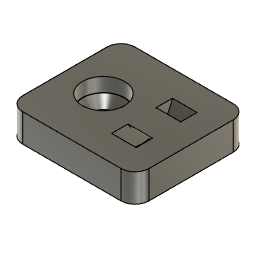
2020 Zip Tie Mount v5 (Autodesk Fusion 360 design; units mm, degrees)
Autodesk Fusion 360 part; units mm, degrees
note: some values were not read from the file. Set by a fixed rule: which sketch regions a step uses.
sketch "Sketch1" plane through (0, 0, 0) normal (0, 0, 1) x (1, 0, 0)
  line L0 (9, 8) -> (-9, 8)
  line L1 (-9, 8) -> (-9, -8)
  line L2 (-9, -8) -> (9, -8)
  line L3 (9, -8) -> (9, 8)
  circle A0 centre (-3.5, 0) radius 1.75
  circle A1 centre (-3.5, 0) radius 3
  line L4 (9, -2.8) -> (-9, -2.8)
  line L5 (-9, -2.8) -> (-9, 2.8)
  line L6 (-9, 2.8) -> (9, 2.8)
  line L7 (9, 2.8) -> (9, -2.8)
  line L8 (9, -2.8) -> (-9, 2.8) construction
  line L9 (-9, -2.8) -> (9, 2.8) construction
  dimension "d1" = 18
  dimension "d2" = 16
  dimension "d5" = 3.5
  dimension "d6" = 6
  dimension "d9" = 5.6
  dimension "d12" = 3.5
  dimension "d23" = 8
  constraint horizontal L0
  constraint perpendicular L0 L1
  constraint parallel L0 L2
  constraint parallel L1 L3
  constraint concentric A0 A1
  constraint horizontal L4
  constraint perpendicular L4 L5
  constraint parallel L4 L6
  constraint parallel L5 L7
  constraint coincident L3 L4.start
  constraint coincident L8 origin
  constraint coincident L9 origin
  constraint horizontal origin A0.centre
  constraint coincident L1 L4.end
  measures "d1" distance of L1.end L2.end
  measures "d2" distance of L0.end L1.end
  measures "d5" diameter of A0
  measures "d6" diameter of A1
  measures "d9" distance of L4 L6
  measures "d12" distance of origin A0.centre
  measures "d23" distance of L0 A0.centre
extrude "Extrude1" add sketch "Sketch1" along normal blind 2
extrude "Extrude2" add sketch "Sketch1" along normal blind 4 contours L0 L1 L3 A1 L6 | L3 A1 L4 L6 L7 | L1 A1 L4 L5 L6 | L1 L2 L3 A1 L4
extrude "Extrude3" add sketch "Sketch1" against normal blind 1 contours L3 A1 L4 L6 L7 | L1 A1 L4 L5 L6 | A1 L4 L6
sketch "Sketch2" plane through (9, 0, 0) normal (1, 0, 0) x (0, 1, 0)
  line L0 (-8, 0) -> (-2.8, 0)
  line L1 (-2.8, 0) -> (-2.8, -1)
  line L2 (-2.8, -1) -> (2.8, -1)
  line L3 (2.8, -1) -> (2.8, 0)
  line L4 (2.8, 0) -> (8, 0)
  line L5 (8, 0) -> (8, 4)
  line L6 (8, 4) -> (-8, 4)
  line L7 (-8, 4) -> (-8, 0)
  circle A0 centre (0, 5) radius 2.25
  circle A1 centre (0, 5) radius 4.45
  line L8 (-8, 0) -> (8, 0)
  line L9 (0, 4) -> (0, 5) construction
  dimension "d13" = 4.5
  dimension "d14" = 2.2
  dimension "d18" = 5
  constraint concentric A0 A1
  constraint midpoint L6 L9.start
  constraint coincident A0.centre A1.centre
  constraint vertical L9
  measures "d13" diameter of A0
  measures "d14" distance of A0 A1
  measures "d18" distance of A0.centre L8
extrude "Extrude4" cut sketch "Sketch2" against normal blind 3.5 from surface at -3.5 contours L6 A0 A1 picked at (-0.2762, 1.3019)
chamfer "Chamfer1" distance 1.2 angle 45 1 edges at (-5.1316, 0.6328, 2)
fillet "Fillet1" radius 2 4 edges at (-9, -8, 2) (9, -8, 2) (9, 8, 2) (-9, 8, 2)
chamfer "Chamfer2" distance 1 angle 45 2 edges at (-9, 0, -1) (9, 0, -1)
equation "d23 = d2 / 2"
